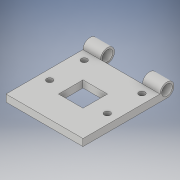
# Autodesk Inventor part: Top of the cam case (real version)
Saved by Autodesk Inventor 2017 (Build 210142000, 142)
## iProperties
Created: 2020-02-10
Part Number: Top of the cam case (real version)
Material: Generic
Document SubType Name: Modeling
Designer: S346559073
Density: 1 g/cm^3
Appearance: Default
Author: S346559073
Autodesk Inventor part; units mm, degrees
ref_plane "YZ Plane" through (0, 0, 0) normal (1, 0, 0) x (0, 1, 0)
ref_plane "XZ Plane" through (0, 0, 0) normal (0, 1, 0) x (-1, 0, 0)
sketch "Sketch1" plane through (0, 0, 0) normal (0, 1, 0) x (-1, 0, 0)
  line L0 (0, 0) -> (27.94, 0)
  line L1 (27.94, 0) -> (27.94, 27.94)
  line L2 (27.94, 27.94) -> (0, 27.94)
  line L3 (0, 27.94) -> (0, 0)
  line L4 (18.415, 18.415) -> (9.525, 18.415)
  line L5 (9.525, 18.415) -> (9.525, 9.525)
  line L6 (9.525, 9.525) -> (18.415, 9.525)
  line L7 (18.415, 9.525) -> (18.415, 18.415)
  line L8 (27.94, 0) -> (18.415, 9.525)
  line L9 (9.525, 18.415) -> (0, 27.94)
  line L10 (27.94, 27.94) -> (18.415, 18.415)
  line L11 (9.525, 9.525) -> (0, 0)
  dimension "d0" = 27.94
  dimension "d1" = 8.89
  constraints: 24 end point, 8 perpendicular, 4 parallel, 2 horizontal
  measures "d0" distance of L2.end L1.end
  measures "d1" distance of L6.end L5.end
extrude "Extrusion1" add sketch "Sketch1" along normal blind 2.54 contours L11 L6 L8 L0 | L3 L9 L5 L11 | L8 L7 L10 L1 | L2 L10 L4 L9
sketch "Sketch2" plane through (0, 0, 27.94) normal (1, 0, 0) x (0, 0, -1)
  circle A0 centre (30.48, 2.54) radius 2.54
  line L0 (27.94, 0) -> (30.48, 0)
  line L1 (27.94, 2.5262) -> (27.94, 0)
  circle A1 centre (30.48, 2.54) radius 1.905
  line L2 (0, 0) -> (27.94, 0) projected
  line L3 (27.94, 0) -> (27.94, 2.54) projected
  line L4 (27.94, 2.54) -> (27.94, 0)
  line L5 (27.94, 0) -> (30.48, 0)
  line L6 (27.94, 2.54) -> (28.575, 2.54)
  line L7 (28.575, 2.54) -> (28.575, 0)
  line L8 (28.575, 0) -> (27.94, 0)
  line L9 (27.94, 0) -> (27.94, 2.54)
  line L10 (30.48, 0.635) -> (27.94, 0.635)
  line L11 (27.94, 0.635) -> (27.94, 0)
  line L12 (27.94, 0) -> (30.48, 0)
  line L13 (30.48, 0) -> (30.48, 0.635)
  line L14 (28.9005, 1.0162) -> (28.3369, 1.0162)
  line L15 (28.3369, 1.0162) -> (28.3369, 0.4026)
  line L16 (28.3369, 0.4026) -> (28.9005, 0.4026)
  line L17 (28.9005, 0.4026) -> (28.9005, 1.0162)
  dimension "d4" = 5.08
  dimension "d5" = 3.81
  constraints: 32 end point, 8 equal length, 6 horizontal, 3 perpendicular, 3 vertical, 2 point on line, 2 vertical alignment, 1 coincident, 1 collinear, 4 other
sketch "Sketch3" plane through (-27.94, 0, 0) normal (-1, 0, 0) x (0, 0, 1)
  circle A0 centre (-2.54, 2.54) radius 1.905
  circle A1 centre (-2.54, 2.54) radius 2.54
  line L0 (-0.3403, 2.54) -> (-0.3403, 0)
  line L1 (0, 2.54) -> (0, 0) projected
  line L2 (-0.3403, 0) -> (0, 0)
  line L3 (0, 0) -> (0, 2.54)
  line L4 (0, 2.54) -> (-0.3403, 2.54)
  line L5 (0, 0) -> (-5.4168, 0)
  line L6 (0, 0) -> (0, 2.54) projected
  line L7 (0, 2.0092) -> (-0.6973, 2.0092)
  line L8 (-0.6973, 2.0092) -> (-0.6973, 0)
  line L9 (-0.6973, 0) -> (0, 0)
  line L10 (0, 0) -> (0, 2.0092)
  line L11 (-2.54, 0.635) -> (0, 0.635)
  line L12 (0, 0.635) -> (0, 0)
  line L13 (0, 0) -> (-2.54, 0)
  line L14 (-2.54, 0) -> (-2.54, 0.635)
  line L15 (-1.27, 1.1201) -> (0, 1.1201)
  line L16 (0, 1.1201) -> (0, 0)
  line L17 (0, 0) -> (-1.27, 0)
  line L18 (-1.27, 0) -> (-1.27, 1.1201)
  point P0 (0, 1.27)
  dimension "d10" = 5.08
  dimension "d11" = 3.81
  constraints: 34 end point, 8 equal length, 5 perpendicular, 4 horizontal, 2 centre point, 2 point on circle, 2 point on line, 2 tangent, 1 coincident, 1 midpoint
  measures "d10" diameter of A1
  measures "d11" diameter of A0
ref_plane "Work Plane1" through (-6.35, 0, 0) normal (0, 0, -1) x (-1, 0, 0)
sketch "Sketch5" plane through (0, 0, 0) normal (0, -1, 0) x (1, 0, 0)
  circle A0 centre (-24.3621, 3.1287) radius 1.0795
  circle A1 centre (-24.3621, 3.1287) radius 1.0795 projected
  circle A2 centre (-3.4325, 3.1287) radius 1.0795
  circle A3 centre (-3.4325, 15.6763) radius 1.0795
  circle A4 centre (-24.3621, 15.6763) radius 1.0795
  circle A5 centre (-3.4325, 15.6763) radius 1.0795
  circle A6 centre (-3.4325, 3.1287) radius 1.0795
  circle A7 centre (-24.3621, 3.1287) radius 1.0795
  circle A8 centre (-24.3621, 15.6763) radius 1.0795
  point P0 (0, 0)
  constraints: 8 centre point, 4 coincident, 3 concentric
extrude "Extrusion5" cut sketch "Sketch5" against normal blind 6.0325
extrude "Extrusion6" add sketch "Sketch2" against normal blind 6.35 contours A0 L13 A1 L6 | L6 L7 L14 A0 | L0 L7 L16 L17 A0 | A0 L17 L10 L13 | A0 L14 L15 L10 L1 | A1 L10 L17 L14 L7 | L17 L16 L7 L10 A0 | A0 L10 L17 | L0 L1 L10 L15 L16 L7 | L14 L7 A0 | A0 L7 L10 L15 L14 | L14 L17 L10 A0 L7 | L10 L7 A0 | L16 L15 L10 L7
extrude "Extrusion7" add sketch "Sketch3" against normal blind 6.35 contours A0 L14 A1 L4 L0 L7 L8 L15 | A0 L18 L11 | L11 L18 A1 L14 | L15 L8 A1 L11 L18 | L11 A1 L18 | A1 L18 L5 | L15 A1 L8 | L8 L7 L0 A1 L15 | L11 L8 L5 L18 A1 | A1 L8 L11 | A1 L7 L0 L4 | A1 L15 L0 L11 L8 | A1 L0 L15 | L11 L0 L5 L8 | L7 L1 L15 L0 A1 | A1 L0 L7 | L15 L1 L11 L0 | L11 L1 L2 L0
body "Solid1"
